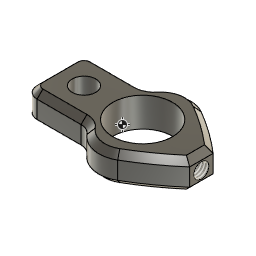
Tuner v3 (Autodesk Fusion 360 design; units mm, degrees)
Autodesk Fusion 360 part; units mm, degrees
sketch "Sketch1" plane through (0, 0, 0) normal (0, 0, 1) x (1, 0, 0)
  circle A0 centre (0, 0) radius 5.08
  line L0 (0, 0) -> (0, -10) construction
  line L1 (0, -10) -> (0, 0) construction
  line L2 (0, 0) -> (0, 10) construction
  line L3 (0, 10) -> (-15, 10)
  line L4 (-15, 10) -> (-15, -10)
  line L5 (-15, -10) -> (10, -10)
  line L6 (10, -10) -> (10, 10)
  line L7 (10, 10) -> (0, 10)
  dimension "d1" = 10.16
  constraint coincident A0.centre L0.start
  constraint vertical L0
  constraint parallel L0 L1
  constraint parallel L0 L2
  constraint perpendicular L2 L3
  constraint perpendicular L3 L4
  constraint perpendicular L0 L5
  constraint perpendicular L3 L6
  constraint perpendicular L2 L7
  measures "d1" diameter of A0
extrude "Extrude1" add sketch "Sketch1" along normal blind 5
sketch "Sketch2" plane through (-15, 0, 0) normal (-1, 0, 0) x (0, -1, 0)
  line L0 (-10, 0) -> (10, 0)
  line L1 (10, 0) -> (10, 5)
  line L2 (10, 5) -> (-10, 5)
  line L3 (-10, 5) -> (-10, 0)
  line L4 (-5, 5) -> (5, 5)
  line L5 (5, 5) -> (5, 0)
  line L6 (5, 0) -> (-5, 0)
  line L7 (-5, 0) -> (-5, 5)
  line L8 (-10, 0) -> (10, 0)
  line L9 (10, 0) -> (10, 5)
  line L10 (10, 5) -> (-10, 5)
  line L11 (-10, 5) -> (-10, 0)
  constraint horizontal L4
  constraint vertical L5
  constraint horizontal L6
  constraint vertical L7
  constraint coincident L2 L4.start
  constraint horizontal L8
  constraint vertical L9
  constraint horizontal L10
  constraint vertical L11
  constraint coincident L1.end L2.start
  constraint coincident L0.start L3.end
extrude "Extrude2" cut sketch "Sketch2" against normal blind 12 contours L0 L2 L3 L7 L8 L10 L11 | L0 L1 L2 L5 L8 L9 L10
fillet "Fillet1" radius 2.5 2 edges at (-3, -5, 2.5) (-3, 5, 2.5)
fillet "Fillet2" radius 2 2 edges at (-15, 5, 2.5) (-15, -5, 2.5)
chamfer "Chamfer1" distance 8 angle 45 2 edges at (10, 10, 2.5) (10, -10, 2.5)
fillet "Fillet3" radius 47 2 edges at (2, -10, 2.5) (2, 10, 2.5)
fillet "Fillet4" radius 5 2 edges at (-3, -10, 2.5) (-3, 10, 2.5)
sketch "Sketch3" plane through (10, 0, 0) normal (1, 0, 0) x (0, 1, 0)
  line L0 (-2, 5) -> (-2, 0)
  line L1 (-2, 0) -> (2, 0)
  line L2 (2, 0) -> (2, 5)
  line L3 (2, 5) -> (-2, 5)
  circle A0 centre (0, 2.5) radius 1.6
  dimension "d18" = 3.2
  measures "d18" diameter of A0
extrude "Extrude4" cut sketch "Sketch3" against normal blind 9 contours A0
thread "Thread1" "ISO Metric profile 3.0 M3x0.5 6H" major diameter 3.086 minor diameter 2.529 pitch 0.5 angle 60 resizes the face on face at (8.2747, -1.5944, 2.6336)
sketch "Sketch4" plane through (0, 0, 5) normal (0, 0, 1) x (-1, 0, 0)
  arc A0 (-2.8559, -7.1128) -> (3.5538, -5.9309) centre (-0.3387, -2.7927) ccw
  arc A1 (5.5, -5) -> (3.5538, -5.9309) centre (5.5, -7.5) ccw
  line L0 (5.5, -5) -> (13, -5)
  arc A2 (13, -5) -> (15, -3) centre (13, -3) ccw
  line L1 (15, -3) -> (15, 3)
  arc A3 (15, 3) -> (13, 5) centre (13, 3) ccw
  line L2 (13, 5) -> (5.5, 5)
  arc A4 (3.5538, 5.9309) -> (5.5, 5) centre (5.5, 7.5) ccw
  arc A5 (3.5538, 5.9309) -> (-2.8559, 7.1128) centre (-0.3387, 2.7927) ccw
  arc A6 (-2.8559, 7.1128) -> (-10, 2) centre (20.8056, -33.4967) ccw
  line L3 (-10, 2) -> (-10, -2)
  arc A7 (-10, -2) -> (-2.8559, -7.1128) centre (20.8056, 33.4967) ccw
  circle A8 centre (0, 0) radius 5.08
  line L4 (15, 0) -> (5.08, 0)
  line L5 (10, 5) -> (10, -5)
  constraint midpoint L1 L4.start
  constraint coincident A8 L4.end
  constraint perpendicular L1 L4
  constraint coincident L2 L5.start
  constraint coincident L0 L5.end
  constraint perpendicular L0 L5
hole "Hole1" at (-9.9982, -0.0032, 5) direction (0, 0, -1) diameter 4 depth 5 tip angle 118
chamfer "Chamfer2" distance 1 angle 45 11 edges at (-9.25, -5, 5) (-4.4213, -5.2447, 5) (-0.568, -7.7098, 5) (6.5477, -4.7237, 5) (6.5477, 4.7237, 5) (-0.568, 7.7098, 5) (-4.4213, 5.2447, 5) (-9.25, 5, 5) (-14.4142, 4.4142, 5) (-15, 0, 5) (-14.4142, -4.4142, 5)
chamfer "Chamfer3" distance 1 angle 45 11 edges at (-9.25, 5, 0) (-4.4213, 5.2447, 0) (-0.568, 7.7098, 0) (6.5477, 4.7237, 0) (6.5477, -4.7237, 0) (-0.568, -7.7098, 0) (-4.4213, -5.2447, 0) (-9.25, -5, 0) (-14.4142, -4.4142, 0) (-15, 0, 0) (-14.4142, 4.4142, 0)
chamfer "Chamfer4" distance 1 angle 45 1 edges at (10, 0, 5)
chamfer "Chamfer5" distance 1 angle 45 1 edges at (10, 0, 0)
